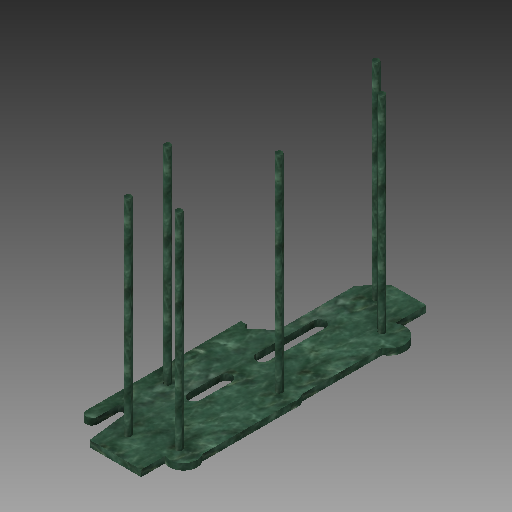
# Autodesk Inventor part: side frame
Saved by Autodesk Inventor 2017 (Build 210142000, 142)
## iProperties
Created: 2019-12-31
Part Number: side frame
Material: Gold
Document SubType Name: Modeling
Designer: Admin
Density: 19.3 g/cm^3
Appearance: Green Polished
Mass: 407.208 g
Surface Area: 182.617 cm^2
Volume: 21.0988 cm^3
Author: Admin
Autodesk Inventor part; units mm, degrees
ref_plane "YZ Plane" through (0, 0, 0) normal (1, 0, 0) x (0, 1, 0)
ref_plane "XZ Plane" through (0, 0, 0) normal (0, 1, 0) x (-1, 0, 0)
ref_plane "XY Plane" through (0, 0, 0) normal (0, 0, 1) x (1, 0, 0)
sketch "Sketch1" plane through (0, 0, 0) normal (0, 1, 0) x (-1, 0, 0)
  line L0 (28.1772, 16.0943) -> (28.1772, -60.1057)
  arc A0 (28.1772, 16.0943) -> (22.6105, 16.0943) centre (25.3938, 16.0943) ccw
  line L1 (22.6105, 16.0943) -> (22.6105, 5.742)
  arc A1 (17.2913, 6.3906) -> (22.6105, 5.742) centre (20.1042, 7.3237) ccw
  line L2 (17.2913, 6.3906) -> (14.6966, 27.8574)
  line L3 (14.6966, 27.8574) -> (-10.7034, 27.8574)
  line L4 (28.1772, -60.1057) -> (25.3938, -60.1057)
  arc A2 (25.3938, -60.1057) -> (21.832, -60.1057) centre (23.6129, -60.0791) ccw
  line L5 (21.832, -60.1057) -> (15.1934, -65.1367)
  line L6 (15.1934, -65.1367) -> (15.1934, -103.2367)
  line L7 (15.1934, -103.2367) -> (6.6122, -112.599)
  line L8 (6.6122, -112.599) -> (-10.7034, -112.599)
  arc A3 (-10.7034, 16.1016) -> (-19.1021, 6.0789) centre (-13.5463, 9.9536) ccw
  arc A4 (-18.0532, -83.5582) -> (-10.7034, -97.3622) centre (-14.3783, -90.4602) ccw
  arc A5 (-19.1021, -37.7307) -> (-18.0532, -44.077) centre (-12.3602, -39.8763) ccw
  line L9 (-10.7034, -97.3622) -> (-10.7034, -112.599)
  line L10 (-18.0532, -44.077) -> (-18.0532, -83.5582)
  line L11 (-10.7034, 27.8574) -> (-10.7034, 16.1016)
  line L12 (-19.1021, 6.0789) -> (-19.1021, -37.7307)
  circle A6 centre (-11.1017, 9.6199) radius 1.5875
  circle A7 centre (-11.1017, -39.6796) radius 1.5875
  circle A8 centre (-11.1017, -90.2764) radius 1.5875
  circle A9 centre (19.7754, -15.645) radius 1.5875
  circle A10 centre (4.4807, -102.9933) radius 1.5875
  line L13 (7.4505, -16.3741) -> (7.4505, -32.0564) construction
  line L14 (4.4666, -16.3741) -> (4.4666, -32.0564)
  line L15 (10.4344, -32.0564) -> (10.4344, -16.3741)
  arc A11 (10.4344, -16.3741) -> (4.4666, -16.3741) centre (7.4505, -16.3741) ccw
  arc A12 (4.4666, -32.0564) -> (10.4344, -32.0564) centre (7.4505, -32.0564) ccw
  line L16 (7.4505, -49.9083) -> (7.4505, -78.16) construction
  line L17 (4.4666, -49.9083) -> (4.4666, -78.16)
  line L18 (10.4344, -78.16) -> (10.4344, -49.9083)
  arc A13 (10.4344, -49.9083) -> (4.4666, -49.9083) centre (7.4505, -49.9083) ccw
  arc A14 (4.4666, -78.16) -> (10.4344, -78.16) centre (7.4505, -78.16) ccw
  circle A15 centre (7.4505, 16.1016) radius 1.5875
  point P0 (0, 0)
  point P1 (7.4505, -24.2152)
  point P2 (7.4505, -64.0341)
  dimension "d0" = 76.2
  dimension "d1" = 25.4
  dimension "d3" = 38.1
  dimension "d4" = 12.7
  dimension "d6" = 3.175
  dimension "d7" = 3.175
  dimension "d8" = 3.175
  dimension "d9" = 3.175
  dimension "d10" = 3.175
  dimension "d11" = 3.175
  constraints: 42 end point, 20 point on circle, 16 centre point, 9 tangent, 8 vertical, 4 perpendicular, 2 horizontal, 2 midpoint, 2 parallel, 2 point on line
  measures "d0" distance of L0.start L0.end
  measures "d1" distance of L2.end L3.end
  measures "d3" distance of L5.end L6.end
  measures "d4" distance of L6.end L7.end
  measures "d6" diameter of A6
  measures "d7" diameter of A7
  measures "d8" diameter of A8
  measures "d9" diameter of A9
  measures "d10" diameter of A10
  measures "d11" diameter of A15
extrude "Extrusion1" add sketch "Sketch1" along normal blind 3.175
sketch "Sketch2" plane through (0, 3.175, 0) normal (0, 1, 0) x (1, 0, 0)
  arc A0 (-10.4344, 49.9083) -> (-4.4666, 49.9083) centre (-7.4505, 49.9083) ccw projected
  line L0 (-10.4344, 49.9083) -> (-10.4344, 78.16) projected
  arc A1 (-4.4666, 78.16) -> (-10.4344, 78.16) centre (-7.4505, 78.16) ccw projected
  line L1 (-4.4666, 78.16) -> (-4.4666, 49.9083) projected
  arc A2 (-10.4344, 16.3741) -> (-4.4666, 16.3741) centre (-7.4505, 16.3741) ccw projected
  line L2 (-10.4344, 16.3741) -> (-10.4344, 32.0564) projected
  arc A3 (-4.4666, 32.0564) -> (-10.4344, 32.0564) centre (-7.4505, 32.0564) ccw projected
  line L3 (-4.4666, 32.0564) -> (-4.4666, 16.3741) projected
  circle A4 centre (-7.4505, -16.1016) radius 1.5875 projected
  circle A5 centre (-4.4807, 102.9933) radius 1.5875 projected
  circle A6 centre (-19.7754, 15.645) radius 1.5875 projected
  circle A7 centre (11.1017, 90.2764) radius 1.5875 projected
  circle A8 centre (11.1017, 39.6796) radius 1.5875 projected
  circle A9 centre (11.1017, -9.6199) radius 1.5875 projected
  line L4 (-28.1772, 60.1057) -> (-28.1772, -16.0943) projected
  arc A10 (-28.1772, -16.0943) -> (-22.6105, -16.0943) centre (-25.3938, -16.0943) ccw projected
  line L5 (-22.6105, -16.0943) -> (-22.6105, -5.742) projected
  arc A11 (-17.2913, -6.3906) -> (-22.6105, -5.742) centre (-20.1042, -7.3237) ccw projected
  line L6 (-17.2913, -6.3906) -> (-14.6966, -27.8574) projected
  line L7 (-14.6966, -27.8574) -> (10.7034, -27.8574) projected
  line L8 (10.7034, -27.8574) -> (10.7034, -16.1016) projected
  arc A12 (10.7034, -16.1016) -> (19.1021, -6.0789) centre (13.5463, -9.9536) ccw projected
  line L9 (19.1021, -6.0789) -> (19.1021, 37.7307) projected
  arc A13 (19.1021, 37.7307) -> (18.0532, 44.077) centre (12.3602, 39.8763) ccw projected
  line L10 (18.0532, 44.077) -> (18.0532, 83.5582) projected
  arc A14 (18.0532, 83.5582) -> (10.7034, 97.3622) centre (14.3783, 90.4602) ccw projected
  line L11 (10.7034, 97.3622) -> (10.7034, 112.599) projected
  line L12 (10.7034, 112.599) -> (-6.6122, 112.599) projected
  line L13 (-6.6122, 112.599) -> (-15.1934, 103.2367) projected
  line L14 (-15.1934, 103.2367) -> (-15.1934, 65.1367) projected
  line L15 (-15.1934, 65.1367) -> (-21.832, 60.1057) projected
  arc A15 (-25.3938, 60.1057) -> (-21.832, 60.1057) centre (-23.6129, 60.0791) ccw projected
  line L16 (-25.3938, 60.1057) -> (-28.1772, 60.1057) projected
  circle A16 centre (-19.7754, 15.645) radius 1.5875
  circle A17 centre (-7.4505, -16.1016) radius 1.5875
  circle A18 centre (11.1017, -9.6199) radius 1.5875
  circle A19 centre (11.1017, 39.6796) radius 1.5875
  circle A20 centre (11.1017, 90.2764) radius 1.5712
  circle A21 centre (-4.4807, 102.9933) radius 1.5875
  point P0 (0, 0)
  constraints: 6 centre point, 6 coincident, 4 concentric
extrude "Extrusion2" add sketch "Sketch2" along normal blind 101.6 contours A4 | A5 | A6 | A8 | A9 | A20
body "Solid1"
